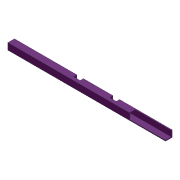
# Autodesk Inventor part: Shovel_CrossFrame
Saved by Autodesk Inventor 2012 (Build 160160000, 160)
## iProperties
Created: 2013-01-29
Part Number: Shovel_CrossFrame
Material: Aluminum-6061
Document SubType Name: Modeling
Designer: JesseK
Density: 2.71 g/cm^3
Mass: 397.252 g
Surface Area: 946.772 cm^2
Volume: 146.587 cm^3
Author: JesseK
Autodesk Inventor part; units mm, degrees
ref_plane "YZ Plane" through (0, 0, 0) normal (1, 0, 0) x (0, 1, 0)
ref_plane "XZ Plane" through (0, 0, 0) normal (0, 1, 0) x (-1, 0, 0)
ref_plane "XY Plane" through (0, 0, 0) normal (0, 0, 1) x (1, 0, 0)
sketch "Sketch1" plane through (0, 0, 0) normal (0, 0, 1) x (1, 0, 0)
  line L0 (0, 0) -> (-609.6, 0)
  line L1 (-609.6, 0) -> (-609.6, 25.4)
  line L2 (-609.6, 25.4) -> (0, 25.4)
  line L3 (0, 25.4) -> (0, 0)
  dimension "d0" = 25.4
  dimension "d1" = 609.6
  constraints: 8 end point, 2 parallel, 1 horizontal, 1 perpendicular
  measures "d0" distance of L2.end L0.start
  measures "d1" distance of L0.start L0.end
extrude "Extrusion1" add sketch "Sketch1" along normal blind 25.4
shell "Shell2" thickness 3.175 removed faces 2 at (-609.6, 8.4667, 16.9333) at (0, 16.9333, 8.4667)
sketch "Sketch3" plane through (0, 0, 25.4) normal (0, 0, 1) x (1, 0, 0)
  line L0 (0, 25.4) -> (-139.7, 25.4)
  line L1 (-139.7, 25.4) -> (-139.7, 3.175)
  line L2 (-139.7, 3.175) -> (0, 3.175)
  line L3 (0, 3.175) -> (0, 25.4)
  dimension "d9" = 22.225
  dimension "d10" = 139.7
  constraints: 8 end point, 2 parallel, 1 horizontal, 1 perpendicular
  measures "d9" distance of L0.end L1.end
  measures "d10" distance of L1.end L2.end
extrude "Extrusion3" cut sketch "Sketch3" against normal blind 22.225
sketch "Sketch4" plane through (-609.6, 0, 0) normal (0, -1, 0) x (1, 0, 0)
  line L0 (361.95, 0) -> (387.35, 0)
  line L1 (387.35, 0) -> (387.35, 12.7)
  line L2 (387.35, 12.7) -> (361.95, 12.7)
  line L3 (361.95, 12.7) -> (361.95, 0)
  line L4 (222.25, 0) -> (247.65, 0)
  line L5 (247.65, 0) -> (247.65, 12.7)
  line L6 (247.65, 12.7) -> (222.25, 12.7)
  line L7 (222.25, 12.7) -> (222.25, 0)
  line L8 (222.25, 0) -> (0, 0) construction
  line L9 (387.35, 0) -> (609.6, 0) construction
  dimension "d13" = 12.7
  dimension "d14" = 25.4
  dimension "d18" = 114.3
  constraints: 20 end point, 4 horizontal, 4 parallel, 3 equal length, 2 perpendicular
  measures "d13" distance of L2.end L0.start
  measures "d14" distance of L1.end L2.end
  measures "d18" distance between parallel lines of L3 L5
extrude "Extrusion4" cut sketch "Sketch4" against normal through all
body "Solid1"
